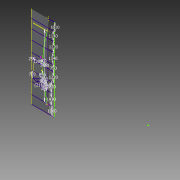
# Autodesk Inventor part: skilt2
Saved by Autodesk Inventor 2015 (Build 190159000, 159)
## iProperties
Created: 2015-09-14
Part Number: skilt2
Material: Generic
Document SubType Name: Modeling
Designer: Simen
Density: 1 g/cm^3
Appearance: Driftwood
Author: Simen
Autodesk Inventor part; units mm, degrees
ref_plane "YZ Plane" through (0, 0, 0) normal (1, 0, 0) x (0, 1, 0)
ref_plane "XZ Plane" through (0, 0, 0) normal (0, 1, 0) x (-1, 0, 0)
ref_plane "XY Plane" through (0, 0, 0) normal (0, 0, 1) x (1, 0, 0)
sketch "Sketch1" plane through (0, 0, 0) normal (0, 1, 0) x (-1, 0, 0)
  line L0 (2004.2593, 9395.4592) -> (-195.7407, 9395.4592)
  line L1 (-195.7407, 9395.4592) -> (-195.7407, -1004.5408)
  line L2 (-195.7407, -1004.5408) -> (2004.2593, -1004.5408)
  line L3 (2004.2593, -1004.5408) -> (2004.2593, 9395.4592)
  point P0 (0, 0)
  dimension "d0" = 2200
  dimension "d1" = 10400
  constraints: 8 end point, 2 parallel, 1 horizontal, 1 perpendicular
  measures "d0" distance of L2.end L1.end
  measures "d1" distance of L1.end L0.end
extrude "Extrusion1" add sketch "Sketch1" along normal blind 12
sketch "L" plane through (0, 12, 0) normal (0, 1, 0) x (1, 0, 0)
  line L0 (-2004.2593, -9395.4592) -> (195.7407, -9395.4592) projected
  line L1 (195.7407, -9395.4592) -> (195.7407, 1004.5408) projected
  line L2 (195.7407, 1004.5408) -> (-2004.2593, 1004.5408) projected
  line L3 (-2004.2593, 1004.5408) -> (-2004.2593, -9395.4592) projected
  line L4 (-2004.2593, -9395.4592) -> (195.7407, -9395.4592) projected
  line L5 (-106.1637, 1004.5408) -> (-106.1637, -95.4592)
  line L6 (-1754.2593, -7995.4592) -> (45.7407, -7995.4592)
  line L7 (-1754.2593, -7995.4592) -> (-1754.2593, -7695.4592)
  line L8 (-1754.2593, -7695.4592) -> (-354.2593, -7695.4592)
  line L9 (-354.2593, -7695.4592) -> (-474.2593, -7215.4592)
  line L10 (-474.2593, -7215.4592) -> (-174.2593, -7215.4592)
  line L11 (-174.2593, -7215.4592) -> (45.7407, -7995.4592)
  line L12 (45.7407, -7995.4592) -> (45.7407, -7215.4592)
  line L13 (152.3488, -8495.1819) -> (932.3488, -8495.1819) construction
  line L14 (45.7407, -7215.4592) -> (-174.2593, -7215.4592)
  line L15 (-1754.2593, -8478.1639) -> (-2004.2593, -8478.1639)
  line L16 (-1343.0832, -7995.4592) -> (-1343.0832, -9395.4592)
  line L17 (-1343.0832, -7995.4592) -> (-1343.0832, -8175.4592)
  line L18 (-324.2593, -7215.4592) -> (-324.2593, -7035.4592)
  point P0 (0, 0)
  dimension "d79" = 1100
  dimension "d89" = 1800
  dimension "d90" = 300
  dimension "d91" = 1400
  dimension "d93" = 300
  dimension "d95" = 90
  dimension "d96" = 220
  dimension "d97" = 250
  dimension "d98" = 1400
  dimension "d204" = 180
  dimension "d206" = 780
  dimension "d207" = 180
  constraints: 28 end point, 6 point on line, 4 horizontal, 4 perpendicular, 2 vertical, 1 midpoint
  measures "d79" distance of L5.start L5.end
  measures "d89" distance of L6.start L6.end
  measures "d90" distance of L6.start L7.end
  measures "d91" distance of L7.end L8.end
  measures "d93" distance of L9.end L10.end
  measures "d95" angle of L13 L12
  measures "d96" distance of L12.end L10.end
  measures "d97" distance of L15.start L15.end
  measures "d98" distance of L16.start L16.end
  measures "d204" distance of L16.start L17.end
  measures "d206" distance of L6.end L12.end
  measures "d207" distance of L18.start L18.end
sketch "U" plane through (0, 12, 0) normal (0, 1, 0) x (1, 0, 0)
  line L0 (-1754.2593, -6995.4592) -> (-1754.2593, -6695.4592)
  line L1 (-1754.2593, -6695.4592) -> (-904.2593, -6695.4592)
  line L2 (-904.2593, -6695.4592) -> (-904.2593, -6145.4592)
  line L3 (-904.2593, -6145.4592) -> (-1754.2593, -6145.4592)
  line L4 (-1754.2593, -6145.4592) -> (-1754.2593, -5845.4592)
  line L5 (-1754.2593, -5845.4592) -> (-904.2593, -5845.4592)
  arc A0 (-904.2593, -6695.4592) -> (-904.2593, -6145.4592) centre (-904.2593, -6420.4592) ccw
  line L6 (-1754.2593, -7695.4592) -> (-354.2593, -7695.4592) projected
  line L7 (-904.2593, -6995.4592) -> (-904.2593, -7695.4592)
  line L8 (-1754.2593, -6878.4482) -> (-2004.2593, -6878.4482)
  line L9 (-2004.2593, 1004.5408) -> (-2004.2593, -9395.4592) projected
  arc A1 (-904.2593, -6995.4592) -> (-904.2593, -5845.4592) centre (-904.2593, -6420.4592) ccw
  line L10 (-1754.2593, -6995.4592) -> (-904.2593, -6995.4592)
  point P0 (0, 0)
  point P1 (-1409.2346, -6695.4592)
  dimension "d99" = 850
  dimension "d100" = 300
  dimension "d101" = 850
  dimension "d102" = 550
  dimension "d103" = 300
  dimension "d104" = 700
  dimension "d105" = 250
  constraints: 18 end point, 7 point on line, 6 perpendicular, 4 point on circle, 2 centre point, 1 coincident, 1 horizontal, 1 vertical
  measures "d99" distance of L0.start L7.start
  measures "d100" distance of L0.start L0.end
  measures "d101" distance of L0.end L1.end
  measures "d102" distance of L1.end L2.end
  measures "d103" distance of L3.end L4.end
  measures "d104" distance of L7.start L7.end
  measures "d105" distance of L8.start L8.end
sketch "R" plane through (0, 12, 0) normal (0, 1, 0) x (1, 0, 0)
  line L0 (-484.2593, -5445.4592) -> (-1754.2593, -5445.4592)
  line L1 (-501.7012, -5145.4592) -> (-634.2593, -5145.4592)
  line L2 (-1754.2593, -5445.4592) -> (-1754.2593, -5145.4592)
  line L3 (-1754.2593, -5845.4592) -> (-854.2593, -5845.4592) projected
  line L4 (-2004.2593, 1004.5408) -> (-2004.2593, -9395.4592) projected
  line L5 (-534.2593, -4585.4592) -> (-752.3018, -4801.55)
  line L6 (-514.9106, -4918.2583) -> (-643.2602, -5045.4592)
  arc A0 (-634.2593, -5145.4592) -> (-1754.2593, -5145.4592) centre (-1194.2593, -5145.4592) ccw
  line L7 (-484.2593, -5445.4592) -> (-501.7012, -5145.4592)
  line L8 (-514.9106, -4918.2583) -> (-534.2593, -4585.4592)
  line L9 (-2004.2593, -9395.4592) -> (195.7407, -9395.4592) projected
  line L10 (195.7407, -9395.4592) -> (195.7407, 1004.5408) projected
  line L11 (195.7407, 1004.5408) -> (-2004.2593, 1004.5408) projected
  line L12 (-2004.2593, 1004.5408) -> (-2004.2593, -9395.4592) projected
  line L13 (-1754.2593, -5145.4592) -> (-1194.2593, -5145.4592)
  line L14 (-1754.2593, -5145.4592) -> (-1194.2593, -5145.4592)
  point P0 (0, 0)
  dimension "d107" = 1270
  dimension "d113" = 300
  dimension "d210" = 300
  dimension "d212" = 50
  dimension "d214" = 250
  dimension "d218" = 400
  dimension "d219" = 1120
  dimension "d220" = 100
  dimension "d221" = 250
  dimension "d223" = 300
  dimension "d224" = 860
  dimension "d225" = 17.4419
  dimension "d226" = 30.6512
  dimension "d227" = 560
  dimension "d228" = 332.7991
  dimension "d229" = 150
  constraints: 18 end point, 5 coincident, 5 point on circle, 4 horizontal, 1 centre point, 1 vertical
  measures "d107" distance of L0.start L0.end
  measures "d113" distance of L2.end L0.end
  measures "d210" distance between parallel lines of L1 L0
  measures "d212" horizontal distance of L5.start L0.start
  measures "d214" distance between parallel lines of L6 L5
  measures "d218" distance between parallel lines of L0 L3
  measures "d219" diameter of A0
  measures "d220" vertical distance of L1.end L6.end
  measures "d221" distance between parallel lines of L4 L2
  measures "d223" distance from line of L0 L13.end
  measures "d224" vertical distance of point (-534.259, -4585.459) L0.start
  measures "d225" horizontal distance of L0.start point (-501.701, -5145.459)
  measures "d226" horizontal distance of L0.start point (-514.911, -4918.258)
  measures "d227" distance of L13.end L2.end
  measures "d228" vertical distance of point (-534.259, -4585.459) point (-514.911, -4918.258)
  measures "d229" horizontal distance of L0.start L1.end
sketch "I" plane through (0, 12, 0) normal (0, 1, 0) x (1, 0, 0)
  line L0 (-1754.2593, -4271.2731) -> (-554.2593, -4271.2731)
  line L1 (-554.2593, -4271.2731) -> (-554.2593, -3971.2731)
  line L2 (-554.2593, -3971.2731) -> (-1754.2593, -3971.2731)
  line L3 (-1754.2593, -3971.2731) -> (-1754.2593, -4271.2731)
  line L4 (-1754.2593, -4121.2731) -> (-2004.2593, -4121.2731)
  line L5 (-2004.2593, 1004.5408) -> (-2004.2593, -9395.4592) projected
  line L6 (-804.2593, -4745.4592) -> (-494.0035, -4642.0405) projected
  line L7 (-484.2593, -4671.2731) -> (-484.2593, -4271.2731)
  line L8 (-554.2593, -4271.2731) -> (-484.2593, -4271.2731)
  point P0 (0, 0)
  dimension "d116" = 1200
  dimension "d117" = 300
  dimension "d118" = 250
  dimension "d119" = 400
  constraints: 14 end point, 5 perpendicular, 1 horizontal, 1 midpoint, 1 point on line, 1 vertical
  measures "d116" distance of L0.start L0.end
  measures "d117" distance of L0.end L1.end
  measures "d118" distance of L4.start L4.end
  measures "d119" distance of L6.end L7.end
sketch "F" plane through (0, 12, 0) normal (0, 1, 0) x (1, 0, 0)
  line L0 (-554.2593, -3971.2731) -> (-1754.2593, -3971.2731) projected
  line L1 (-1754.2593, -3621.2731) -> (-544.2593, -3621.2731)
  line L2 (-544.2593, -3621.2731) -> (-534.2593, -3321.4398)
  line L3 (-534.2593, -3321.4398) -> (-754.2593, -3321.4398)
  line L4 (-754.2593, -3321.4398) -> (-754.2593, -2821.4398)
  line L5 (-754.2593, -2821.4398) -> (-1054.2593, -2821.4398)
  line L6 (-1054.2593, -2821.4398) -> (-1054.2593, -3321.2731)
  line L7 (-1054.2593, -3321.2731) -> (-1454.2593, -3321.2731)
  line L8 (-1454.2593, -3321.2731) -> (-1454.2593, -2671.2731)
  line L9 (-1454.2593, -2671.2731) -> (-1754.2593, -2671.2731)
  line L10 (-1754.2593, -2671.2731) -> (-1754.2593, -3621.2731)
  line L11 (-1754.2593, -3971.2731) -> (-1754.2593, -4271.2731) projected
  line L12 (-1754.2593, -3254.3076) -> (-2004.2593, -3254.3076)
  line L13 (-2004.2593, 1004.5408) -> (-2004.2593, -9395.4592) projected
  line L14 (-1303.0158, -3621.2731) -> (-1303.0158, -3971.2731)
  line L15 (-1238.9692, -3321.2731) -> (-1238.9692, -3621.2731)
  line L16 (-2004.2593, -9395.4592) -> (195.7407, -9395.4592) projected
  line L17 (195.7407, -9395.4592) -> (195.7407, 1004.5408) projected
  line L18 (195.7407, 1004.5408) -> (-2004.2593, 1004.5408) projected
  line L19 (-2004.2593, 1004.5408) -> (-2004.2593, -9395.4592) projected
  point P0 (0, 0)
  dimension "d120" = 1210
  dimension "d121" = 300
  dimension "d122" = 220
  dimension "d123" = 500
  dimension "d124" = 300
  dimension "d125" = 400
  dimension "d126" = 650
  dimension "d127" = 300
  dimension "d128" = 250
  dimension "d129" = 350
  dimension "d130" = 300
  constraints: 26 end point, 7 perpendicular, 6 point on line, 2 horizontal, 2 parallel, 1 vertical
  measures "d120" distance of L1.start L1.end
  measures "d121" distance of L1.end L2.end
  measures "d122" distance of L2.end L3.end
  measures "d123" distance of L3.end L4.end
  measures "d124" distance of L4.end L5.end
  measures "d125" distance of L6.end L7.end
  measures "d126" distance of L7.end L8.end
  measures "d127" distance of L8.end L9.end
  measures "d128" distance of L12.start L12.end
  measures "d129" distance of L14.start L14.end
  measures "d130" distance of L15.start L15.end
sketch "A" plane through (0, 12, 0) normal (0, 1, 0) x (1, 0, 0)
  line L0 (-464.2593, -2471.4398) -> (-294.2593, -2471.4398)
  line L1 (-294.2593, -2471.4398) -> (-294.2593, -1371.4398)
  line L2 (-294.2593, -1371.4398) -> (-464.2593, -2471.4398)
  line L3 (-1754.2593, -2671.2731) -> (-1754.2593, -3621.2731) projected
  line L4 (-1454.2593, -2671.2731) -> (-1754.2593, -2671.2731) projected
  line L5 (-1754.2593, -2671.2731) -> (-1754.2593, -1971.2731)
  line L6 (-1754.2593, -1971.2731) -> (-464.2593, -2471.4398)
  line L7 (-294.2593, -1371.4398) -> (-1754.2593, -1971.2731)
  line L8 (-544.2593, -3621.2731) -> (-534.2593, -3321.4398) projected
  line L9 (-534.2593, -3321.4398) -> (-754.2593, -3321.4398) projected
  line L10 (-464.2593, -2471.4398) -> (-418.4397, -2174.9595)
  line L11 (-418.4397, -2174.9595) -> (-604.9137, -2102.6586)
  line L12 (-604.9137, -2102.6586) -> (-551.1272, -1754.6281)
  line L13 (-294.2593, -1371.4398) -> (-340.079, -1667.9201)
  line L14 (-340.079, -1667.9201) -> (-551.1272, -1754.6281)
  line L15 (-1754.2593, -7995.4592) -> (45.7407, -7995.4592) projected
  line L16 (45.7407, -7995.4592) -> (45.7407, -95.4592)
  line L17 (-534.2593, -3321.4398) -> (-534.2593, -2471.4398)
  line L18 (-534.2593, -2471.4398) -> (-464.2593, -2471.4398)
  line L19 (-418.4397, -2174.9595) -> (-410.803, -2125.5461)
  line L20 (-604.9137, -2102.6586) -> (-1360.7491, -1809.6015)
  line L21 (-1360.7491, -1809.6015) -> (-1754.2593, -1971.2731)
  line L22 (-551.1272, -1754.6281) -> (-1406.5688, -2106.0818)
  point P0 (0, 0)
  dimension "d137" = 170
  dimension "d138" = 1100
  dimension "d139" = 700
  dimension "d141" = 300
  dimension "d142" = 200
  dimension "d144" = 300
  dimension "d147" = 7900
  dimension "d186" = 850
  dimension "d187" = 70
  dimension "d188" = 50
  dimension "d254" = 211.0482
  constraints: 36 end point, 5 parallel, 5 point on line, 3 vertical, 1 collinear, 1 horizontal, 1 perpendicular
  measures "d137" distance of L0.start L0.end
  measures "d138" distance of L0.end L1.end
  measures "d139" distance of L3.start L5.end
  measures "d141" distance of L0.start L10.end
  measures "d142" distance of L10.end L11.end
  measures "d144" distance of L1.end L13.end
  measures "d147" distance of L15.end L16.end
  measures "d186" distance of L8.end L17.end
  measures "d187" distance of L17.end L0.start
  measures "d188" distance of L10.end L19.end
  measures "d254" horizontal distance of L13.end L12.end
sketch "X" plane through (0, 12, 0) normal (0, 1, 0) x (1, 0, 0)
  line L0 (-294.2593, -1371.4398) -> (-1754.2593, -1971.2731) projected
  line L1 (-294.2593, -2471.4398) -> (-294.2593, -1371.4398) projected
  line L2 (45.7407, -7995.4592) -> (45.7407, -95.4592) projected
  line L3 (-64.2593, -466.3883) -> (45.7407, -95.4592)
  line L4 (-1754.2593, -1971.2731) -> (-1754.2593, 739.9844)
  line L5 (-262.203, -1264.8378) -> (-188.0155, -958.2141)
  line L6 (-1754.2593, -346.224) -> (-1270.1203, -644.2937)
  line L7 (-955.3825, -838.0683) -> (-262.203, -1264.8378)
  line L8 (-1754.2593, -846.224) -> (-1270.1203, -644.2937)
  line L9 (-928.9972, -502.0141) -> (45.7407, -95.4592)
  line L10 (-1754.2593, -1171.2731) -> (-955.3825, -838.0683)
  line L11 (-614.2593, -695.7887) -> (-64.2593, -466.3883)
  line L12 (-188.0155, -958.2141) -> (-614.2593, -695.7887)
  line L13 (-928.9972, -502.0141) -> (-1754.2593, 6.0748)
  line L14 (-2004.2593, -9395.4592) -> (195.7407, -9395.4592) projected
  line L15 (195.7407, -9395.4592) -> (195.7407, 1004.5408) projected
  line L16 (195.7407, 1004.5408) -> (-2004.2593, 1004.5408) projected
  line L17 (-2004.2593, 1004.5408) -> (-2004.2593, -9395.4592) projected
  line L18 (45.7407, -95.4592) -> (195.7407, -95.4592)
  line L19 (-64.2593, -466.3883) -> (45.7407, -420.5082)
  line L20 (45.7407, -95.4592) -> (-1754.2593, -95.4592)
  line L21 (-262.203, -1264.8378) -> (45.7407, -1454.4294)
  line L22 (-188.0155, -958.2141) -> (45.7407, -1102.1306)
  point P0 (-1754.2593, -1221.2731)
  dimension "d242" = 110
  dimension "d243" = 800
  dimension "d245" = 500
  dimension "d246" = 550
  dimension "d247" = 300
  dimension "d248" = 300
  dimension "d252" = 150
  dimension "d253" = 325.0491
  dimension "d255" = 250.7649
  dimension "d256" = 325.0491
  dimension "d257" = 352.2988
  dimension "d261" = 681.6224
  dimension "d262" = 352.2988
  constraints: 32 end point, 9 point on line, 7 parallel, 5 collinear, 2 perpendicular, 1 vertical
  measures "d242" distance from line of L2 L3.start
  measures "d243" distance of L10.start L0.end
  measures "d245" distance of L6.start L8.start
  measures "d246" horizontal distance of L3.start L11.start
  measures "d247" distance between parallel lines of L13 L6
  measures "d248" distance between parallel lines of L10 L8
  measures "d252" distance of L2.end L18.end
  measures "d253" distance of L2.end L19.end
  measures "d255" distance of L20.end L6.start
  measures "d256" distance of L8.start L10.start
  measures "d257" distance of L13.end L6.start
  measures "d261" distance of L22.end L19.end
  measures "d262" distance of L21.end L22.end
sketch "Moduler" plane through (0, 12, 0) normal (0, 1, 0) x (1, 0, 0)
  line L0 (195.7407, -9395.4592) -> (933.3112, -9395.4592)
  line L1 (933.3112, -9395.4592) -> (933.3112, -8385.4592)
  line L2 (933.3112, -8385.4592) -> (-2004.2593, -8385.4592)
  line L3 (933.3112, -8385.4592) -> (933.3112, -7245.4592)
  line L4 (933.3112, -7245.4592) -> (-2004.2593, -7245.4592)
  line L5 (933.3112, -7245.4592) -> (933.3112, -6025.4592)
  line L6 (933.3112, -6025.4592) -> (-2004.2593, -6025.4592)
  line L7 (-2004.2593, 1004.5408) -> (-2004.2593, -9395.4592) projected
  line L8 (933.3112, -6025.4592) -> (933.3112, -4685.4592)
  line L9 (933.3112, -4685.4592) -> (-2004.2593, -4685.4592)
  line L10 (933.3112, -4685.4592) -> (933.3112, -3935.4592)
  line L11 (933.3112, -3935.4592) -> (-2004.2593, -3935.4592)
  line L12 (933.3112, -3935.4592) -> (933.3112, -2715.4592)
  line L13 (933.3112, -2715.4592) -> (-2004.2593, -2715.4592)
  line L14 (933.3112, -2715.4592) -> (933.3112, -1495.4592)
  line L15 (933.3112, -1495.4592) -> (-2004.2593, -1495.4592)
  line L16 (933.3112, -1495.4592) -> (933.3112, -85.4592)
  line L17 (933.3112, -85.4592) -> (-2004.2593, -85.4592)
  line L18 (933.3112, -85.4592) -> (933.3112, 974.5408)
  line L19 (933.3112, 974.5408) -> (-2004.2593, 974.5408)
  point P0 (0, 0)
  dimension "d150" = 1010
  dimension "d151" = 1140
  dimension "d152" = 1220
  dimension "d153" = 1340
  dimension "d154" = 750
  dimension "d155" = 1220
  dimension "d157" = 1410
  dimension "d222" = 1060
  dimension "d263" = 1220
  constraints: 38 end point, 11 point on line, 10 perpendicular, 3 vertical, 1 horizontal
  measures "d150" distance of L0.end L1.end
  measures "d151" distance of L1.end L3.end
  measures "d152" distance of L3.end L5.end
  measures "d153" distance of L5.end L8.end
  measures "d154" distance of L8.end L10.end
  measures "d155" distance of L10.end L12.end
  measures "d157" distance of L14.end L16.end
  measures "d222" distance of L16.end L18.end
  measures "d263" distance between parallel lines of L15 L13
extrude "Extrusion2" add sketch "L" along normal blind 100 contours L6 L7 L8 L9 L10 L11
extrude "Extrusion3" add sketch "U" along normal blind 100 contours L0 L1 A0 L3 L4 L5 A1 L10
extrude "Extrusion5" add sketch "I" along normal blind 100
extrude "Extrusion6" add sketch "F" along normal blind 100 contours L10 L9 L8 L7 L15 L1 | L15 L7 L6 L5 L4 L3 L2 L1
extrude "Extrusion7" add sketch "A" along normal blind 100 contours L6 L22 L20 L11 L2 | L6 L7 L20 L22 | L2 L14 L22 L20 L7 | L20 L22 L12
sketch "Sketch14" plane through (0, 12, 0) normal (0, 1, 0) x (1, 0, 0)
  arc A0 (45.7407, -95.4592) -> (45.7407, -7995.4592) centre (12745.7407, -4045.4592) ccw
  point P0 (0, 0)
  constraints: 2 point on circle, 1 centre point
extrude "Extrusion10" add sketch "R" along normal blind 100 contours L0 L2 A0 L1 L7 | L5 L8 L6 A0
extrude "Extrusion11" add sketch "X" along normal blind 100 contours L7 L10 L4 L8 L6 L20 L13 L9 L3 L11 L12 L5 | L20 L4 L13
body "Solid1"
